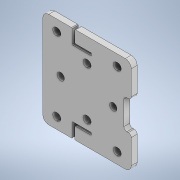
# Autodesk Inventor part: podstawa_lewa
Saved by Autodesk Inventor 2020 (Build 240168000, 168)
## iProperties
Created: 2020-09-29
Part Number: podstawa_lewa
Material: Ogólny
Document SubType Name: Konstrukcja blachowa
Designer: szymo
Density: 1 g/cm^3
Sheet Metal Rule: Domyślny_mm
Appearance: Domyślna
Author: szymo
Autodesk Inventor part; units mm, degrees
ref_plane "YZ Plane" through (0, 0, 0) normal (1, 0, 0) x (0, 1, 0)
ref_plane "XZ Plane" through (0, 0, 0) normal (0, 1, 0) x (-1, 0, 0)
ref_plane "XY Plane" through (0, 0, 0) normal (0, 0, 1) x (1, 0, 0)
sketch "Szkic1" plane through (0, 0, 0) normal (0, 0, 1) x (1, 0, 0)
  line L0 (0, 61) -> (0, 4)
  line L1 (57, 42.5) -> (58, 42.5)
  line L2 (58, 22.5) -> (57, 22.5)
  line L3 (55, 24.5) -> (55, 40.5)
  line L4 (60, 4) -> (60, 20.5)
  line L5 (60, 44.5) -> (60, 61)
  line L6 (4, 0) -> (19.5, 0)
  line L7 (20, 0.5) -> (20, 9.5)
  line L8 (20.5, 10) -> (32.5, 10)
  line L9 (33, 9.5) -> (33, 8.75)
  line L10 (32.5, 8.25) -> (22.25, 8.25)
  line L11 (21.75, 7.75) -> (21.75, 0.5)
  line L12 (0, 0) -> (20, 0)
  line L13 (22.25, 0) -> (56, 0)
  arc A0 (22.25, 8.25) -> (21.75, 7.75) centre (22.25, 7.75) ccw
  arc A1 (20.5, 10) -> (20, 9.5) centre (20.5, 9.5) ccw
  arc A2 (33, 9.5) -> (32.5, 10) centre (32.5, 9.5) ccw
  arc A3 (32.5, 8.25) -> (33, 8.75) centre (32.5, 8.75) ccw
  arc A4 (19.5, 0) -> (20, 0.5) centre (19.5, 0.5) ccw
  arc A5 (21.75, 0.5) -> (22.25, 0) centre (22.25, 0.5) ccw
  arc A6 (60, 20.5) -> (58, 22.5) centre (58, 20.5) ccw
  arc A7 (55, 24.5) -> (57, 22.5) centre (57, 24.5) ccw
  arc A8 (57, 42.5) -> (55, 40.5) centre (57, 40.5) ccw
  arc A9 (58, 42.5) -> (60, 44.5) centre (58, 44.5) ccw
  arc A10 (60, 61) -> (56, 65) centre (56, 61) ccw
  arc A11 (4, 65) -> (0, 61) centre (4, 61) ccw
  arc A12 (0, 4) -> (4, 0) centre (4, 4) ccw
  arc A13 (56, 0) -> (60, 4) centre (56, 4) ccw
  line L14 (20, 64.5) -> (20, 55.5)
  line L15 (20.5, 55) -> (32.5, 55)
  line L16 (33, 55.5) -> (33, 56.25)
  line L17 (32.5, 56.75) -> (22.25, 56.75)
  line L18 (21.75, 57.25) -> (21.75, 64.5)
  arc A14 (21.75, 57.25) -> (22.25, 56.75) centre (22.25, 57.25) ccw
  arc A15 (20, 55.5) -> (20.5, 55) centre (20.5, 55.5) ccw
  arc A16 (32.5, 55) -> (33, 55.5) centre (32.5, 55.5) ccw
  arc A17 (33, 56.25) -> (32.5, 56.75) centre (32.5, 56.25) ccw
  arc A18 (20, 64.5) -> (19.5, 65) centre (19.5, 64.5) ccw
  arc A19 (22.25, 65) -> (21.75, 64.5) centre (22.25, 64.5) ccw
  circle A20 centre (47.85, 32.5) radius 2.5
  line L19 (56, 65) -> (22.25, 65)
  line L20 (19.5, 65) -> (4, 65)
  arc A21 (9.25, 60) -> (9.25, 55) centre (9.25, 57.5) ccw
  arc A22 (9.75, 55) -> (9.75, 60) centre (9.75, 57.5) ccw
  line L21 (9.25, 60) -> (9.75, 60)
  line L22 (9.25, 55) -> (9.75, 55)
  arc A23 (30.25, 46.5) -> (30.25, 51.5) centre (30.25, 49) ccw
  arc A24 (29.75, 51.5) -> (29.75, 46.5) centre (29.75, 49) ccw
  line L23 (29.75, 51.5) -> (30.25, 51.5)
  line L24 (29.75, 46.5) -> (30.25, 46.5)
  line L25 (9.85, 32.5) -> (9.6, 32.5)
  line L26 (9.6, 32.5) -> (10.1, 32.5)
  circle A25 centre (12.15, 32.5) radius 2.5
  arc A26 (50.75, 55) -> (50.75, 60) centre (50.75, 57.5) ccw
  arc A27 (50.25, 60) -> (50.25, 55) centre (50.25, 57.5) ccw
  line L27 (50.75, 60) -> (50.25, 60)
  line L28 (50.75, 55) -> (50.25, 55)
  arc A28 (9.25, 10) -> (9.25, 5) centre (9.25, 7.5) ccw
  arc A29 (9.75, 5) -> (9.75, 10) centre (9.75, 7.5) ccw
  line L29 (9.25, 5) -> (9.75, 5)
  line L30 (9.25, 10) -> (9.75, 10)
  arc A30 (30.25, 13.5) -> (30.25, 18.5) centre (30.25, 16) ccw
  arc A31 (29.75, 18.5) -> (29.75, 13.5) centre (29.75, 16) ccw
  line L31 (29.75, 13.5) -> (30.25, 13.5)
  line L32 (29.75, 18.5) -> (30.25, 18.5)
  arc A32 (50.25, 10) -> (50.25, 5) centre (50.25, 7.5) ccw
  line L33 (50.75, 10) -> (50.25, 10)
  arc A33 (50.75, 5) -> (50.75, 10) centre (50.75, 7.5) ccw
  line L34 (50.75, 5) -> (50.25, 5)
  point P0 (60, 65)
  point P1 (60, 0)
  point P2 (0, 65)
  point P3 (60, 22.5)
  point P4 (60, 42.5)
  point P5 (55, 22.5)
  point P6 (20, 10)
  point P7 (33, 10)
  point P8 (33, 8.25)
  point P9 (21.75, 8.25)
  dimension "d0" = 60
  dimension "d1" = 65
  dimension "d4" = 5
  dimension "d5" = 20
  dimension "d6" = 20
  dimension "d7" = 10
  dimension "d8" = 13
  dimension "d9" = 1.75
  dimension "d10" = 11.25
  dimension "d11" = 0.5
  dimension "d12" = 2
  dimension "d13" = 4
  dimension "d21" = 9.85
  dimension "d22" = 5
  dimension "d23" = 38
  dimension "d29" = 5
  dimension "d30" = 5
  dimension "d33" = 5
  dimension "d34" = 5
  dimension "d36" = 0.25
  dimension "d37" = 0.5
  measures "d0" distance of point (0, 65) point (60, 65)
  measures "d1" distance of point (60, 65) point (60, 0)
  measures "d4" distance of point (60, 22.5) point (55, 22.5)
  measures "d5" distance of point (60, 42.5) point (60, 22.5)
  measures "d6" distance of L12.start L12.end
  measures "d7" distance of L12.end point (20, 10)
  measures "d8" distance of point (20, 10) point (33, 10)
  measures "d9" distance of point (33, 10) point (33, 8.25)
  measures "d10" distance of point (33, 8.25) point (21.75, 8.25)
  measures "d11" radius of A0
  measures "d12" radius of A6
  measures "d13" radius of A10
  measures "d21" distance from line of L0 L25.start
  measures "d22" diameter of A20
  measures "d23" distance of L25.start A20.centre
  measures "d29" diameter of A21
  measures "d30" diameter of A22
  measures "d33" diameter of A23
  measures "d34" diameter of A24
  measures "d36" distance of L25.start L25.end
  measures "d37" distance of L25.end L26.end
extrude "Płyta2" add sketch "Szkic1" along normal blind 4
equation "\"d40\" = Grubość"
equation "\"PromieńGięcia\" = Grubość"
equation "\"SzerokośćGięciaPodcięcia\" = Grubość"
equation "\"GłębokośćGięciaPodcięcia\" = 0.5 * Grubość"
equation "\"RozmiarPodcięciaNarożnika\" = 4 * Grubość"
equation "\"MinimalnaPozostałość\" = 2 * Grubość"
equation "\"PromieńPrzejścia\" = PromieńGięcia"
equation "\"Rozmiar_promienia_Jacobiego\" = PromieńGięcia"
equation "\"Wielk_odstępu\" = Grubość"
equation "\"Grubość\" = 4"
